fixed jaw v1 (Autodesk Fusion 360 design; units mm, degrees)
Autodesk Fusion 360 part; units mm, degrees
sketch "Sketch1" plane through (0, 0, 0) normal (0, 0, 1) x (1, 0, 0)
  line L0 (160, -190) -> (-160, -190)
  line L1 (-160, -190) -> (-160, 190)
  line L2 (-160, 190) -> (160, 190)
  line L3 (160, 190) -> (160, -190)
  line L4 (160, -190) -> (-160, 190) construction
  line L5 (-160, -190) -> (160, 190) construction
  dimension "d1" = 320
  dimension "d2" = 380
  constraint horizontal L0
  constraint perpendicular L0 L1
  constraint parallel L0 L2
  constraint parallel L1 L3
  constraint coincident L4 origin
  constraint coincident L5 origin
  measures "d1" distance of L1.end L2.end
  measures "d2" distance of L0.end L1.end
extrude "Extrude1" add sketch "Sketch1" along normal blind 25
sketch "Sketch2" plane through (0, 0, 25) normal (0, 0, 1) x (1, 0, 0)
  line L0 (160, 190) -> (-160, 190)
  line L1 (-160, 190) -> (-160, -190)
  line L2 (-160, -190) -> (160, -190)
  line L3 (160, -190) -> (160, 190)
  line L4 (-160, 190) -> (-125, 190)
  line L5 (-125, 190) -> (-125, 170)
  line L6 (-125, 170) -> (-160, 170)
  line L7 (-160, 170) -> (-160, 190)
  line L8 (160, 190) -> (125, 190)
  line L9 (125, 190) -> (125, 170)
  line L10 (125, 170) -> (160, 170)
  line L11 (160, 170) -> (160, 190)
  line L12 (160, -190) -> (125, -190)
  line L13 (125, -190) -> (125, -170)
  line L14 (125, -170) -> (160, -170)
  line L15 (160, -170) -> (160, -190)
  line L16 (-160, -190) -> (-125, -190)
  line L17 (-125, -190) -> (-125, -170)
  line L18 (-125, -170) -> (-160, -170)
  line L19 (-160, -170) -> (-160, -190)
  dimension "d5" = 35
  dimension "d6" = 20
  dimension "d7" = 35
  dimension "d8" = 20
  dimension "d9" = 20
  dimension "d10" = 35
  dimension "d11" = 35
  dimension "d12" = 20
  constraint horizontal L4
  constraint vertical L5
  constraint horizontal L6
  constraint vertical L7
  constraint coincident L0.end L1.start
  constraint horizontal L8
  constraint vertical L9
  constraint horizontal L10
  constraint vertical L11
  constraint coincident L0.start L3.end
  constraint horizontal L12
  constraint vertical L13
  constraint horizontal L14
  constraint vertical L15
  constraint coincident L2.end L3.start
  constraint horizontal L16
  constraint vertical L17
  constraint horizontal L18
  constraint vertical L19
  constraint coincident L1.end L2.start
  measures "d5" distance of L17.end L18.end
  measures "d6" distance of L16.end L17.end
  measures "d7" distance of L13.end L14.end
  measures "d8" distance of L12.end L13.end
  measures "d9" distance of L8.end L9.end
  measures "d10" distance of L9.end L10.end
  measures "d11" distance of L5.end L6.end
  measures "d12" distance of L4.end L5.end
hole "Hole1" at (-125, 170, 25) at (125, 170, 25) at (125, -170, 25) at (-125, -170, 25) direction (0, 0, -1) diameter 30 depth 25 tip angle 118
hole "Hole2" at (0, 0, 25) direction (0, 0, -1) diameter 40 depth 50 tip angle 118 counterbore diameter 70 counterbore depth 12
